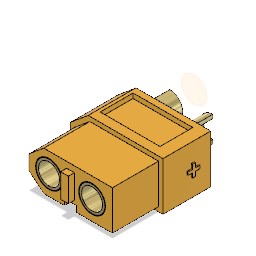
AMASS_XT60-F_1x02_P7.2mm_Vertical (Autodesk Fusion 360 design; units mm, degrees)
Autodesk Fusion 360 part; units mm, degrees
note: some values were not read from the file. Chosen so that the rebuilt part matches the saved one: which bodies a step acts on.
sketch "Sketch1" plane through (0, 0, 0) normal (0, 0, 1) x (1, 0, 0)
  line L0 (0, 0) -> (0, 12.5)
  line L1 (0, 0) -> (8.1, 0)
  line L2 (8.1, 0) -> (8.1, 12.5)
  line L3 (8.1, 12.5) -> (8.1, 15.5) construction
  line L4 (8.1, 15.5) -> (5.6, 15.5) construction
  line L5 (8.1, 12.5) -> (5.6, 15.5)
  line L6 (5.6, 15.5) -> (2.5, 15.5)
  line L7 (2.5, 15.5) -> (0, 12.5)
  dimension "d1" = 12.5
  dimension "d2" = 8.1
  dimension "d3" = 2.5
  dimension "d4" = 3.1
  constraint coincident L0.start L1.start
  constraint vertical L0
  constraint perpendicular L0 L1
  constraint perpendicular L1 L2
  constraint perpendicular L1 L3
  constraint perpendicular L3 L4
  constraint perpendicular L2 L6
  measures "d1" distance of L0.start L0.end
  measures "d2" distance of L0.start L1.end
  measures "d3" distance of L3.end L4.end
  measures "d4" distance of L4.end L6.end
extrude "Extrude1" add sketch "Sketch1" along normal blind 8 makes body 1
sketch "Sketch2" plane through (0, 0, 8) normal (0, 0, 1) x (1, 0, 0)
  line L0 (0, 0) -> (8.1, 0)
  line L1 (8.1, 0) -> (8.1, 12.5)
  line L2 (8.1, 12.5) -> (5.6, 15.5)
  line L3 (5.6, 15.5) -> (2.5, 15.5)
  line L4 (2.5, 15.5) -> (0, 12.5)
  line L5 (0, 12.5) -> (0, 0)
  line L6 (0.75, 0.75) -> (7.35, 0.75)
  line L7 (7.35, 0.75) -> (7.35, 12.2285)
  line L8 (7.35, 12.2285) -> (5.2487, 14.75)
  line L9 (5.2487, 14.75) -> (2.8513, 14.75)
  line L10 (2.8513, 14.75) -> (0.75, 12.2285)
  line L11 (0.75, 12.2285) -> (0.75, 0.75)
  dimension "d7" = 0.75
extrude "Extrude2" add sketch "Sketch2" along normal blind 7.7 contours L6 L7 L8 L9 L10 L11 bodies 1
sketch "Sketch3" plane through (0.75, 0, 0) normal (-1, 0, 0) x (0, 0, 1)
  line L0 (8, 12.2285) -> (8, 0.75)
  line L1 (8, 0.75) -> (15.7, 0.75)
  line L2 (15.7, 0.75) -> (15.7, 12.2285)
  line L3 (15.7, 12.2285) -> (8, 12.2285)
  line L4 (15.7, 0.75) -> (15.7, 6.75) construction
  line L5 (15.7, 6.75) -> (8, 6.75)
  line L6 (8, 6.75) -> (8, 8.75)
  line L7 (8, 8.75) -> (15.7, 8.75)
  line L8 (15.7, 8.75) -> (15.7, 6.75)
  dimension "d10" = 6
  dimension "d11" = 2
  constraint coincident L1.end L2.start
  constraint perpendicular L1 L4
  constraint horizontal L5
  constraint vertical L6
  constraint horizontal L7
  constraint vertical L8
  measures "d10" distance of L1.end L4.end
  measures "d11" distance of L4.end L7.end
extrude "Extrude3" cut sketch "Sketch3" against normal blind 1 contours L0 L2 L5 L6 L7 L8 bodies 1
sketch "Sketch4" plane through (0, 0, 15.7) normal (0, 0, 1) x (1, 0, 0)
  line L0 (0.75, 8.75) -> (1.75, 8.75)
  line L1 (1.75, 8.75) -> (1.75, 6.75)
  line L2 (1.75, 6.75) -> (0.75, 6.75)
  line L3 (0.75, 6.75) -> (0.75, 0.75)
  line L4 (0.75, 0.75) -> (7.35, 0.75)
  line L5 (7.35, 0.75) -> (7.35, 12.2285)
  line L6 (7.35, 12.2285) -> (5.2487, 14.75)
  line L7 (5.2487, 14.75) -> (2.8513, 14.75)
  line L8 (2.8513, 14.75) -> (0.75, 12.2285)
  line L9 (0.75, 12.2285) -> (0.75, 8.75)
  line L10 (1.75, 7.75) -> (7.35, 7.7517) construction
  line L11 (6.35, 8.4014) -> (2.35, 8.4014)
  line L12 (2.35, 8.4014) -> (2.35, 7.1014)
  line L13 (2.35, 7.1014) -> (6.35, 7.1014)
  line L14 (6.35, 7.1014) -> (6.35, 8.4014)
  point P0 (1.75, 7.75)
  point P1 (6.35, 7.7514)
  dimension "d14" = 1
  dimension "d15" = 4
  dimension "d16" = 1.3
  constraint midpoint L1 P0
  constraint coincident P0 L10.start
  constraint coincident L5 L10.end
  constraint coincident L10 P1
  constraint horizontal L11
  constraint vertical L12
  constraint horizontal L13
  constraint vertical L14
  constraint midpoint P1 L14
  measures "d14" horizontal distance of L10.end P1
  measures "d15" distance of L11.start L11.end
  measures "d16" distance of L11.start L13.end
extrude "Extrude4" add sketch "Sketch4" along normal blind 1 contours L11 L12 L13 L14 bodies 1
sketch "Sketch5" plane through (0, 0, 0) normal (0, 0, -1) x (-1, 0, 0)
  line L0 (-8.1, 0) -> (0, 0)
  line L1 (0, 0) -> (0, 12.5)
  line L2 (0, 12.5) -> (-2.5, 15.5)
  line L3 (-2.5, 15.5) -> (-5.6, 15.5)
  line L4 (-5.6, 15.5) -> (-8.1, 12.5)
  line L5 (-8.1, 12.5) -> (-8.1, 0)
  line L6 (-4.05, 11.35) -> (-4.05, 15.5) construction
  line L7 (-4.05, 4.15) -> (-4.05, 0) construction
  circle A0 centre (-4.05, 11.35) radius 3
  circle A1 centre (-4.05, 4.15) radius 3
  point P0 (-4.05, 11.35)
  point P1 (-4.05, 4.15)
  dimension "d19" = 7.2
  dimension "d20" = 6
  dimension "d21" = 6
  constraint coincident P0 L6.start
  constraint midpoint L3 L6.end
  constraint perpendicular L3 L6
  constraint coincident P1 L7.start
  constraint midpoint L0 L7.end
  constraint perpendicular L0 L7
  constraint equal L6 L7
  measures "d19" distance of P0 P1
  measures "d20" diameter of A0
  measures "d21" diameter of A1
extrude "Extrude5" cut sketch "Sketch5" against normal blind 3 contours A0 | A1 bodies 1
sketch "Sketch6" plane through (0, 0, 3) normal (0, 0, -1) x (-1, 0, 0)
  circle A0 centre (-4.05, 11.35) radius 3
  circle A1 centre (-4.05, 11.35) radius 2.15
  dimension "d24" = 4.3
  constraint concentric A0 A1
  measures "d24" diameter of A1
sketch "Sketch8" plane through (0, 0, 3) normal (0, 0, -1) x (-1, 0, 0)
  circle A0 centre (-4.05, 4.15) radius 3
  circle A1 centre (-4.05, 4.15) radius 2.15
  dimension "d25" = 4.3
  constraint concentric A0 A1
  measures "d25" diameter of A1
extrude "Extrude6" add sketch "Sketch8" sketch "Sketch6" along normal blind 7.5 contours A1 of sketch 2 contours A1 bodies 1
sketch "Sketch9" plane through (0, 0, -4.5) normal (0, 0, -1) x (-1, 0, 0)
  circle A0 centre (-4.05, 4.15) radius 2.15
hole "Hole1" at (4.05, 4.15, -4.5) direction (0, 0, 1) diameter 3 depth 6 tip angle 118 bodies 1
hole "Hole3" at (4.05, 11.35, -4.5) direction (0, 0, 1) diameter 3 depth 6 tip angle 118 bodies 1
ref_plane "WorkPlane2" through (6.2, 4.15, -0.75) normal (1, 0, 0) x (0, -1, 0)
sketch "Sketch11" plane through (6.2, 4.15, -0.75) normal (1, 0, 0) x (0, 0, -1)
  line L0 (3.75, 0) -> (0.75, 0)
  line L1 (0.75, 0) -> (0.75, -2.2)
  line L2 (0.75, -2.2) -> (3.75, -2.2)
  line L3 (3.75, -2.2) -> (3.75, 0)
  point P0 (3.75, 0)
  dimension "d38" = 3
  constraint horizontal L0
  constraint vertical L1
  constraint horizontal L2
  constraint vertical L3
  constraint coincident P0 L0.start
  measures "d38" distance of P0 L0.end
extrude "Extrude7" cut sketch "Sketch11" against normal blind 5.5 bodies 1
sketch "Sketch12" plane through (6.2, 4.15, -0.75) normal (1, 0, 0) x (0, 0, -1)
  line L0 (3.75, 7.2) -> (0.75, 7.2)
  line L1 (0.75, 7.2) -> (0.75, 9.9)
  line L2 (0.75, 9.9) -> (3.75, 9.9)
  line L3 (3.75, 9.9) -> (3.75, 7.2)
  point P0 (3.75, 7.2)
  dimension "d41" = 3
  constraint horizontal L0
  constraint vertical L1
  constraint horizontal L2
  constraint vertical L3
  constraint coincident P0 L0.start
  measures "d41" distance of P0 L0.end
extrude "Extrude8" cut sketch "Sketch12" against normal blind 6.8 bodies 1
sketch "Sketch13" plane through (0, 0, 15.7) normal (0, 0, 1) x (1, 0, 0)
  line L0 (6.35, 7.1014) -> (2.35, 7.1014)
  line L1 (2.35, 7.1014) -> (2.35, 8.4014)
  line L2 (2.35, 8.4014) -> (6.35, 8.4014)
  line L3 (6.35, 8.4014) -> (6.35, 7.1014)
  line L4 (0.75, 8.75) -> (1.75, 8.75)
  line L5 (1.75, 8.75) -> (1.75, 6.75)
  line L6 (1.75, 6.75) -> (0.75, 6.75)
  line L7 (0.75, 6.75) -> (0.75, 0.75)
  line L8 (0.75, 0.75) -> (7.35, 0.75)
  line L9 (7.35, 0.75) -> (7.35, 12.2285)
  line L10 (7.35, 12.2285) -> (5.2487, 14.75)
  line L11 (5.2487, 14.75) -> (2.8513, 14.75)
  line L12 (2.8513, 14.75) -> (0.75, 12.2285)
  line L13 (0.75, 12.2285) -> (0.75, 8.75)
  circle A0 centre (4.05, 11.35) radius 2.25
  circle A1 centre (4.05, 4.15) radius 2.25
  dimension "d44" = 4.5
  dimension "d45" = 4.5
  measures "d44" diameter of A0
  measures "d45" diameter of A1
extrude "Extrude9" cut sketch "Sketch13" against normal blind 10 contours A0 | A1 bodies 1
sketch "Sketch14" plane through (0, 0, 5.7) normal (0, 0, 1) x (1, 0, 0)
  circle A0 centre (4.05, 4.15) radius 2.25
  circle A1 centre (4.05, 4.15) radius 2.15
  circle A2 centre (4.05, 11.35) radius 2.15
  dimension "d48" = 4.3
  dimension "d49" = 4.3
  constraint concentric A0 A1
  measures "d48" diameter of A1
  measures "d49" diameter of A2
extrude "Extrude10" add sketch "Sketch14" along normal blind 10 contours A1 | A2 bodies 1
hole "Hole4" at (4.05, 11.35, 15.7) direction (0, 0, -1) diameter 3.5 depth 10 tip angle 118 bodies 1
hole "Hole5" at (4.05, 4.15, 15.7) direction (0, 0, -1) diameter 3.5 depth 10 tip angle 118 bodies 1
split "Split1" by face at (6.1973, 11.2428, 12.3667) of body 1 bodies 1 makes body 2 at (6.2972, 4.0378, 9.0333)
split "Split2" by face at (6.1973, 4.0428, 12.3667) of body 2 bodies 2 makes body 3 at (6.2972, 4.0378, 9.0333)
sketch "Sketch15" plane through (0, 15.5, 0) normal (0, 1, 0) x (-1, 0, 0)
  line L0 (-5.6, 0) -> (-2.5, 0)
  line L1 (-2.5, 0) -> (-2.5, 8)
  line L2 (-2.5, 8) -> (-5.6, 8)
  line L3 (-5.6, 8) -> (-5.6, 0)
  line L4 (-4, 0) -> (-4, 3) construction
  line L5 (-5, 3) -> (-3, 3)
  line L6 (-3, 3) -> (-3, 3.2)
  line L7 (-3, 3.2) -> (-5, 3.2)
  line L8 (-5, 3.2) -> (-5, 3)
  dimension "d58" = 3
  dimension "d59" = 2
  dimension "d60" = 0.2
  constraint coincident L0 L4.start
  constraint horizontal L5
  constraint vertical L6
  constraint horizontal L7
  constraint vertical L8
  constraint midpoint L4.end L5
  measures "d58" distance of L4.start L4.end
  measures "d59" distance of L6.end L7.end
  measures "d60" distance of L5.start L7.end
extrude "Extrude11" add sketch "Sketch15" along normal blind 0.2 contours L5 L6 L7 L8 bodies 3
sketch "Sketch16" plane through (0, 0, 0) normal (0, -1, 0) x (1, 0, 0)
  line L0 (0, 0) -> (8.1, 0)
  line L1 (8.1, 0) -> (8.1, 8)
  line L2 (8.1, 8) -> (0, 8)
  line L3 (0, 8) -> (0, 0)
  line L4 (4, 0) -> (4, 2) construction
  line L5 (3.75, 2) -> (4.25, 2)
  line L6 (4.25, 2) -> (4.25, 2.75)
  line L7 (4.25, 2.75) -> (5, 2.75)
  line L8 (5, 2.75) -> (5, 3.25)
  line L9 (5, 3.25) -> (4.25, 3.25)
  line L10 (4.25, 3.25) -> (4.25, 4)
  line L11 (4.25, 4) -> (3.75, 4)
  line L12 (3.75, 4) -> (3.75, 3.25)
  line L13 (3.75, 3.25) -> (3, 3.25)
  line L14 (3, 3.25) -> (3, 2.75)
  line L15 (3, 2.75) -> (3.75, 2.75)
  line L16 (3.75, 2.75) -> (3.75, 2)
  dimension "d63" = 2
  dimension "d64" = 0.5
  dimension "d65" = 0.75
  constraint vertical L4
  constraint coincident L0 L4.start
  constraint perpendicular L1 L5
  constraint perpendicular L5 L6
  constraint perpendicular L1 L7
  constraint perpendicular L5 L8
  constraint perpendicular L1 L9
  constraint perpendicular L9 L10
  constraint perpendicular L1 L11
  constraint perpendicular L11 L12
  constraint perpendicular L12 L13
  constraint perpendicular L13 L14
  constraint perpendicular L14 L15
  constraint perpendicular L15 L16
  constraint equal L15 L16
  constraint equal L6 L7
  constraint equal L6 L16
  constraint equal L7 L9
  constraint equal L9 L10
  constraint equal L10 L12
  constraint equal L12 L13
  constraint equal L13 L15
  constraint equal L11 L14
  constraint equal L5 L14
  constraint equal L5 L8
  constraint midpoint L4.end L5
  measures "d63" distance of L4.start L4.end
  measures "d64" distance of L7.end L8.end
  measures "d65" distance of L8.end L9.end
extrude "Extrude12" add sketch "Sketch16" along normal blind 0.2 contours L5 L6 L7 L8 L9 L10 L11 L12 L13 L14 L15 L16 bodies 3
sketch "Sketch17" plane through (0, 0, 0) normal (-1, 0, 0) x (0, 0, 1)
  line L0 (0, 12.5) -> (0, 0)
  line L1 (0, 0) -> (8, 0)
  line L2 (8, 0) -> (8, 12.5)
  line L3 (8, 12.5) -> (0, 12.5)
  line L4 (1, 0) -> (1, 2) construction
  line L5 (1, 2) -> (0, 2) construction
  line L6 (1, 2) -> (6.5, 2)
  line L7 (6.5, 2) -> (6.5, 12)
  line L8 (6.5, 12) -> (1, 12)
  line L9 (1, 12) -> (1, 2)
  dimension "d68" = 1
  dimension "d69" = 2
  dimension "d70" = 5.5
  dimension "d71" = 10
  constraint coincident L1 L4.start
  constraint perpendicular L1 L4
  constraint coincident L0 L5.end
  constraint horizontal L6
  constraint vertical L7
  constraint horizontal L8
  constraint vertical L9
  measures "d68" distance of L4.end L5.end
  measures "d69" distance of L4.start L4.end
  measures "d70" distance of L4.end L6.end
  measures "d71" distance of L4.end L8.end
extrude "Extrude13" cut sketch "Sketch17" against normal blind 0.8 contours L6 L7 L8 L9 bodies 3
sketch "Sketch18" plane through (8.1, 0, 0) normal (1, 0, 0) x (0, 0, -1)
  line L0 (0, 0) -> (0, 12.5)
  line L1 (0, 12.5) -> (-8, 12.5)
  line L2 (-8, 12.5) -> (-8, 0)
  line L3 (-8, 0) -> (0, 0)
  line L4 (-1, 0) -> (-1, 2) construction
  line L5 (-1, 2) -> (0, 2) construction
  line L6 (-1, 2) -> (-6.5, 2)
  line L7 (-6.5, 2) -> (-6.5, 12)
  line L8 (-6.5, 12) -> (-1, 12)
  line L9 (-1, 12) -> (-1, 2)
  dimension "d74" = 1
  dimension "d75" = 2
  dimension "d76" = 5.5
  dimension "d77" = 10
  constraint coincident L3 L4.start
  constraint perpendicular L3 L4
  constraint coincident L0 L5.end
  constraint perpendicular L0 L5
  constraint horizontal L6
  constraint vertical L7
  constraint horizontal L8
  constraint vertical L9
  measures "d74" distance of L4.end L5.end
  measures "d75" distance of L4.start L4.end
  measures "d76" distance of L4.end L6.end
  measures "d77" distance of L4.end L8.end
extrude "Extrude14" cut sketch "Sketch18" against normal blind 0.8 contours L6 L7 L8 L9 bodies 3
move_body "Move1" bodies 3 2 1 to x (0, 1, 0) y (-1, 0, 0) z (0, 0, 1) at (0, 0, 0)
move_body "Move2" bodies 3 2 1 to x (1, 0, 0) y (0, 1, 0) z (0, 0, 1) at (11.35, -4.05, 0)
named bodies: "Pin 1", "Pin 2", "Body"
